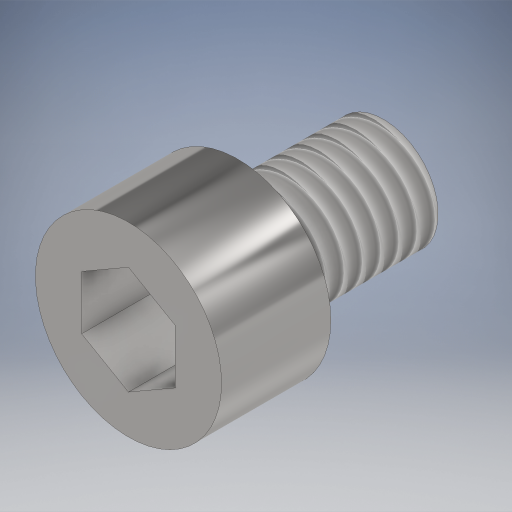
# Autodesk Inventor part: Болт М6
Saved by Autodesk Inventor 2023 (Build 270158000, 158)
## iProperties
Created: 2023-01-04
Part Number: Болт М6
Material: Типовые
Document SubType Name: Modeling
Designer: Admin
Density: 1 g/cm^3
Appearance: По умолчанию
Author: Admin
Autodesk Inventor part; units mm, degrees
ref_plane "YZ Plane" through (0, 0, 0) normal (1, 0, 0) x (0, 1, 0)
ref_plane "XZ Plane" through (0, 0, 0) normal (0, 1, 0) x (-1, 0, 0)
ref_plane "XY Plane" through (0, 0, 0) normal (0, 0, 1) x (1, 0, 0)
sketch "Эскиз1" plane through (0, 0, 0) normal (0, 0, 1) x (1, 0, 0)
  circle A0 centre (0, 0) radius 5.11
  circle A1 centre (0, 0) radius 3
  line L0 (0, 2.9676) -> (2.57, 1.4838)
  line L1 (2.57, 1.4838) -> (2.57, -1.4838)
  line L2 (2.57, -1.4838) -> (0, -2.9676)
  line L3 (0, -2.9676) -> (-2.57, -1.4838)
  line L4 (-2.57, -1.4838) -> (-2.57, 1.4838)
  line L5 (-2.57, 1.4838) -> (0, 2.9676)
  dimension "d0" = 5.14
  dimension "d1" = 10.22
  dimension "d2" = 6
  constraints: 12 end point, 3 coincident, 2 centre point, 1 vertical, 13 other
  measures "d0" distance between parallel lines of L4 L1
  measures "d1" diameter of A0
  measures "d2" diameter of A1
extrude "Выдавливание1" add sketch "Эскиз1" against normal blind 6 contours A0 | A1 | L0 L1 L2 L3 L4 L5
extrude "Выдавливание2" cut sketch "Эскиз1" against normal blind 4 contours L0 L1 L2 L3 L4 L5
sketch "Эскиз2" plane through (0, 0, -6) normal (0, 0, -1) x (-1, 0, 0)
  circle A0 centre (0, 0) radius 3 projected
extrude "Выдавливание3" add sketch "Эскиз2" along normal blind 8
thread "Резьба1" size "M6x1" class "6g" standard "ISO Metric profile" full length
